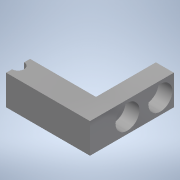
# Autodesk Inventor part: Gripper arm
Saved by Autodesk Inventor 2021 (Build 250183000, 183)
## iProperties
Company: SDU
Created: 2020-11-04
Part Number: Gripper arm
Engr Approved By: Approved By
Material: Steel
Description: Description
Document SubType Name: Modeling
Designer: Kling
Engineer: Engineer
Stock Number: Stock number
Density: 7.85 g/cm^3
Appearance: Steel
RM. Dwg. No.: 5674
RM. File Name: N.A.
RM. No.: 4789
Title: Title
Author: Kling
Autodesk Inventor part; units mm, degrees
ref_plane "YZ Plane" through (0, 0, 0) normal (1, 0, 0) x (0, 1, 0)
ref_plane "XZ Plane" through (0, 0, 0) normal (0, 1, 0) x (-1, 0, 0)
ref_plane "XY Plane" through (0, 0, 0) normal (0, 0, 1) x (1, 0, 0)
sketch "Sketch1" plane through (0, 0, 0) normal (0, 0, 1) x (1, 0, 0)
  line L0 (0, 20) -> (6, 20)
  line L1 (6, 20) -> (6, 0)
  line L2 (6, 0) -> (0, 0)
  line L3 (0, 0) -> (0, 20)
  line L4 (6, 0) -> (-22, 0)
  line L5 (-22, 0) -> (-22, -8)
  line L6 (-22, -8) -> (6, -8)
  line L7 (6, -8) -> (6, 0)
  circle A0 centre (-22, -4) radius 2
  point P0 (0, 0)
  point P1 (-22, -2)
  point P2 (-22, -6)
  dimension "d0" = 20
  dimension "d1" = 6
  dimension "d2" = 4
  dimension "d3" = 8
  dimension "d4" = 22
  constraints: 16 end point, 4 parallel, 2 coincident, 2 horizontal, 2 perpendicular, 1 centre point, 1 midpoint
  measures "d0" distance of L2.end L0.start
  measures "d1" distance of L0.start L0.end
  measures "d2" diameter of A0
  measures "d3" distance of L4.end L5.end
  measures "d4" distance between parallel lines of L3 L5
extrude "Extrusion1" add sketch "Sketch1" along normal blind 10 contours L0 L1 L2 L3 | L2 L7 L6 L5 A0 L4
sketch "Sketch2" plane through (6, -8, 0) normal (1, 0, 0) x (0, 0, -1)
  line L0 (0, 28) -> (-10, 28) projected
  point P0 (0, 8)
  point P1 (-5, 12.5)
  point P2 (-5, 23.5)
  point P3 (-5, 28)
  dimension "d14" = 11
  dimension "d15" = 4.5
  constraints: 2 vertical alignment, 1 midpoint
  measures "d14" distance of point (-5, 12.5) point (-5, 23.5)
  measures "d15" distance of point (-5, 28) point (-5, 23.5)
hole "Hole1" at (6, 15.5, 5) at (6, 4.5, 5) direction (-1, 0, 0) diameter 4.5 end through all counterbore diameter 8 counterbore depth 4.6 clearance for "Socket Head Cap Screw ISO 4762" size "M4" standard "ISO"
body "Solid1"
